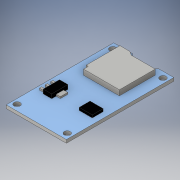
# Autodesk Inventor part: MicroSD Card Reader
Saved by Autodesk Inventor 2016 (Build 200138000, 138)
## iProperties
Created: 2015-11-27
Part Number: MicroSD Card Reader
Material: Generic
Document SubType Name: Modeling
Designer: Spooner
Density: 1 g/cm^3
Appearance: Default
Author: Spooner
Autodesk Inventor part; units mm, degrees
ref_plane "YZ Plane" through (0, 0, 0) normal (1, 0, 0) x (0, 1, 0)
ref_plane "XZ Plane" through (0, 0, 0) normal (0, 1, 0) x (-1, 0, 0)
ref_plane "XY Plane" through (0, 0, 0) normal (0, 0, 1) x (1, 0, 0)
sketch "Sketch1" plane through (0, 0, 0) normal (0, 1, 0) x (-1, 0, 0)
  line L0 (0, 0) -> (-23.5077, 0)
  line L1 (-23.5077, 0) -> (-23.5077, -41.9735)
  line L2 (0, -41.9735) -> (0, 0)
  line L3 (-7.4041, -41.9735) -> (-8.8011, -40.5765)
  line L4 (-8.8011, -40.5765) -> (-16.3322, -40.5765)
  line L5 (-16.3322, -40.5765) -> (-17.7292, -41.9735)
  line L6 (-23.5077, -41.9735) -> (-17.7292, -41.9735)
  line L7 (-7.4041, -41.9735) -> (0, -41.9735)
  circle A0 centre (-1.9431, -39.6748) radius 1.1811
  circle A1 centre (-21.5646, -39.6748) radius 1.1811
  circle A2 centre (-21.5646, -2.2987) radius 1.1811
  circle A3 centre (-1.9431, -2.2987) radius 1.1811
  dimension "d0" = 135
  dimension "d1" = 41.9735
  dimension "d2" = 23.5077
  dimension "d3" = 1.397
  dimension "d4" = 5.7785
  dimension "d5" = 7.4041
  dimension "d6" = 2.3622
  dimension "d7" = 1.1176
  dimension "d8" = 0.762
  dimension "d9" = 0.762
  dimension "d10" = 1.1176
  constraints: 16 end point, 4 centre point, 3 equal radius, 3 horizontal alignment, 3 parallel, 2 horizontal, 2 perpendicular, 2 vertical alignment
  measures "d0" angle of L4 L3
  measures "d1" distance of L2.start L0.start
  measures "d2" distance of L0.start L0.end
  measures "d3" distance between parallel lines of L4 L6
  measures "d4" distance of L1.end L5.end
  measures "d5" distance of L3.start L2.start
  measures "d6" diameter of A0
  measures "d7" distance edge to line of A1 L6
  measures "d8" distance edge to line of A1 L1
  measures "d9" distance edge to line of A0 L2
  measures "d10" distance edge to line of A2 L0
extrude "Extrusion1" add sketch "Sketch1" along normal blind 1.2446
sketch "Sketch2" plane through (0, 1.2446, 0) normal (0, 1, 0) x (1, 0, 0)
  line L0 (9.7028, 39.1795) -> (19.0627, 39.1795)
  line L1 (19.0627, 39.1795) -> (19.0627, 25.146)
  line L2 (19.0627, 25.146) -> (5.08, 25.146)
  line L3 (4.2418, 26.9875) -> (4.2418, 40.1955)
  line L4 (4.2418, 40.1955) -> (8.0518, 40.1955)
  line L5 (8.0518, 40.1955) -> (9.7028, 39.1795)
  line L6 (5.08, 25.146) -> (5.08, 26.9875)
  line L7 (16.3322, 40.5765) -> (8.8011, 40.5765) projected
  line L8 (0, 41.9735) -> (0, 0) projected
  line L9 (4.2418, 26.9875) -> (5.08, 26.9875)
  line L10 (7.4041, 41.9735) -> (0, 41.9735) projected
  point P0 (4.6609, 26.9875)
  dimension "d13" = 14.0335
  dimension "d14" = 1.397
  dimension "d15" = 14.8209
  dimension "d16" = 4.2418
  dimension "d17" = 5.08
  dimension "d18" = 13.208
  dimension "d20" = 1.778
  dimension "d21" = 9.3599
  dimension "d22" = 3.81
  constraints: 16 end point, 2 horizontal, 2 perpendicular, 1 horizontal alignment, 1 midpoint, 1 parallel, 1 vertical
  measures "d13" distance between parallel lines of L2 L0
  measures "d14" distance between parallel lines of L0 L7
  measures "d15" distance between parallel lines of L1 L3
  measures "d16" distance between parallel lines of L8 L3
  measures "d17" distance between parallel lines of L8 L6
  measures "d18" distance of L3.start L3.end
  measures "d20" distance between parallel lines of L4 L10
  measures "d21" distance from line of L0.start L1
  measures "d22" distance of L3.end L4.end
extrude "Extrusion2" add sketch "Sketch2" along normal blind 2.032
sketch "Sketch3" plane through (8.0518, 1.2446, -40.1955) normal (0, 0, -1) x (-1, 0, 0)
  line L0 (-10.1473, 1.778) -> (1.143, 1.778)
  line L1 (1.143, 1.778) -> (1.143, 1.0414)
  line L2 (1.143, 1.0414) -> (-10.1473, 1.0414)
  line L3 (-10.1473, 1.0414) -> (-10.1473, 1.778)
  line L4 (2.9718, 2.032) -> (-11.0109, 2.032) projected
  line L5 (-8.2804, -1.2446) -> (-0.7493, -1.2446) projected
  line L6 (-11.0109, 0) -> (-11.0109, 2.032) projected
  line L7 (3.81, 0) -> (3.81, 2.032) projected
  point P0 (8.0518, -1.2446)
  dimension "d25" = 0.254
  dimension "d26" = 2.286
  dimension "d27" = 0.8636
  dimension "d28" = 2.667
  constraints: 8 end point, 2 parallel, 1 horizontal, 1 perpendicular
  measures "d25" distance between parallel lines of L4 L0
  measures "d26" distance between parallel lines of L5 L2
  measures "d27" distance from line of L6 L0.start
  measures "d28" distance between parallel lines of L7 L1
extrude "Extrusion3" cut sketch "Sketch3" against normal blind 12.192
sketch "Sketch4" plane through (0, 1.2446, 0) normal (0, 1, 0) x (1, 0, 0)
  line L0 (3.5179, 10.9474) -> (6.8199, 10.9474)
  line L1 (6.8199, 10.9474) -> (6.8199, 17.3228)
  line L2 (6.8199, 17.3228) -> (3.5179, 17.3228)
  line L3 (3.5179, 17.3228) -> (3.5179, 10.9474)
  line L4 (5.08, 25.146) -> (19.0627, 25.146) projected
  line L5 (0, 41.9735) -> (0, 0) projected
  dimension "d31" = 6.3754
  dimension "d32" = 3.302
  dimension "d33" = 7.8232
  dimension "d34" = 3.5179
  constraints: 8 end point, 2 parallel, 1 horizontal, 1 perpendicular
  measures "d31" distance of L2.end L0.start
  measures "d32" distance of L1.end L2.end
  measures "d33" distance between parallel lines of L4 L2
  measures "d34" distance between parallel lines of L5 L3
extrude "Extrusion4" add sketch "Sketch4" along normal blind 1.6002
sketch "Sketch5" plane through (0, 1.2446, 0) normal (0, 1, 0) x (1, 0, 0)
  line L0 (3.5179, 10.9474) -> (3.5179, 17.3228) projected
  line L1 (1.4859, 16.764) -> (3.5179, 16.764)
  line L2 (3.5179, 16.764) -> (3.5179, 15.875)
  line L3 (3.5179, 15.875) -> (1.4859, 15.875)
  line L4 (1.4859, 15.875) -> (1.4859, 16.764)
  line L5 (1.4859, 14.5796) -> (3.5179, 14.5796)
  line L6 (3.5179, 14.5796) -> (3.5179, 13.6906)
  line L7 (3.5179, 13.6906) -> (1.4859, 13.6906)
  line L8 (1.4859, 13.6906) -> (1.4859, 14.5796)
  line L9 (1.4859, 12.3952) -> (3.5179, 12.3952)
  line L10 (3.5179, 12.3952) -> (3.5179, 11.5062)
  line L11 (3.5179, 11.5062) -> (1.4859, 11.5062)
  line L12 (1.4859, 11.5062) -> (1.4859, 12.3952)
  line L13 (3.5179, 17.3228) -> (3.5179, 10.9474) projected
  line L14 (6.8199, 17.3228) -> (6.8199, 10.9474) projected
  line L15 (6.8199, 15.5765) -> (8.4709, 15.5765)
  line L16 (8.4709, 15.5765) -> (8.4709, 12.6936)
  line L17 (8.4709, 12.6936) -> (6.8199, 12.6936)
  line L18 (6.8199, 12.6936) -> (6.8199, 15.5765)
  point P0 (0, 0)
  point P1 (1.4859, 14.1351)
  point P2 (3.5179, 14.1351)
  point P3 (8.4709, 14.1351)
  dimension "d37" = 0.889
  dimension "d38" = 2.032
  dimension "d39" = 5.2578
  dimension "d40" = 1.2954
  dimension "d41" = 1.2954
  dimension "d44" = 2.8829
  dimension "d45" = 1.651
  constraints: 32 end point, 8 parallel, 6 point on line, 4 horizontal, 4 perpendicular, 3 midpoint, 2 collinear, 2 horizontal alignment
  measures "d37" distance of L3.end L1.start
  measures "d38" distance of point (3.518, 14.135) point (1.486, 14.135)
  measures "d39" distance between parallel lines of L11 L1
  measures "d40" distance between parallel lines of L5 L3
  measures "d41" distance between parallel lines of L9 L7
  measures "d44" distance of L15.end L16.end
  measures "d45" distance from line of L14 point (8.471, 14.135)
extrude "Extrusion5" add sketch "Sketch5" along normal blind 0.635
sketch "Sketch6" plane through (0, 1.2446, 0) normal (0, 1, 0) x (1, 0, 0)
  line L0 (16.129, 16.637) -> (21.2598, 16.637)
  line L1 (21.2598, 16.637) -> (21.2598, 12.3698)
  line L2 (21.2598, 12.3698) -> (16.129, 12.3698)
  line L3 (16.129, 12.3698) -> (16.129, 16.637)
  line L4 (23.5077, 0) -> (23.5077, 41.9735) projected
  line L5 (5.08, 25.146) -> (19.0627, 25.146) projected
  point P0 (0, 0)
  dimension "d46" = 5.1308
  dimension "d47" = 4.2672
  dimension "d48" = 2.2479
  dimension "d49" = 8.509
  constraints: 8 end point, 2 parallel, 1 horizontal, 1 perpendicular
  measures "d46" distance of L0.start L0.end
  measures "d47" distance of L0.end L1.end
  measures "d48" distance between parallel lines of L4 L1
  measures "d49" distance between parallel lines of L5 L0
extrude "Extrusion6" add sketch "Sketch6" along normal blind 1.016
equation "\"d9\" = d8"
equation "\"d10\" = d7"
equation "\"d40\" = d41"
body "Solid1"
